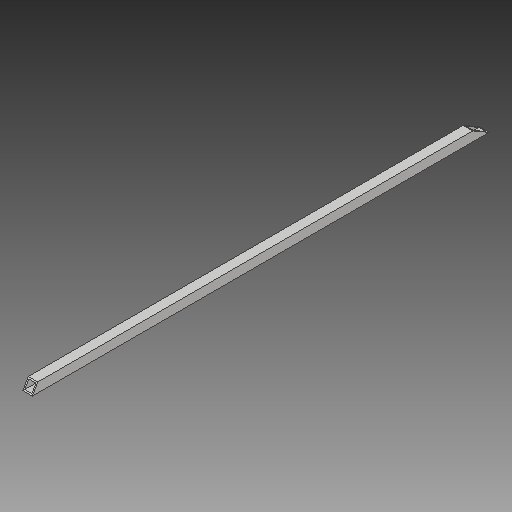
# Autodesk Inventor part: 30-60-supportBrace
Saved by Autodesk Inventor 2018.2 (Build 222227000, 227)
## iProperties
Created: 2018-02-07
Part Number: 30-60-supportBrace
Material: Generic
Document SubType Name: Modeling
Designer: steele
Density: 1 g/cm^3
Appearance: Default
Author: steele
Autodesk Inventor part; units mm, degrees
ref_plane "YZ Plane" through (0, 0, 0) normal (1, 0, 0) x (0, 1, 0)
ref_plane "XZ Plane" through (0, 0, 0) normal (0, 1, 0) x (-1, 0, 0)
ref_plane "XY Plane" through (0, 0, 0) normal (0, 0, 1) x (1, 0, 0)
sketch "Sketch1" plane through (0, 0, 0) normal (0, 0, 1) x (1, 0, 0)
  line L0 (-12.7, -12.7) -> (12.7, -12.7)
  line L1 (12.7, -12.7) -> (12.7, 12.7)
  line L2 (12.7, 12.7) -> (-12.7, 12.7)
  line L3 (-12.7, 12.7) -> (-12.7, -12.7)
  line L4 (-12.7, -12.7) -> (12.7, 12.7) construction
  line L5 (12.7, -12.7) -> (-12.7, 12.7) construction
  line L6 (-9.525, -9.525) -> (9.525, -9.525)
  line L7 (9.525, -9.525) -> (9.525, 9.525)
  line L8 (9.525, 9.525) -> (-9.525, 9.525)
  line L9 (-9.525, 9.525) -> (-9.525, -9.525)
  line L10 (-9.525, -9.525) -> (9.525, 9.525) construction
  line L11 (9.525, -9.525) -> (-9.525, 9.525) construction
  point P0 (0, 0)
  dimension "d0" = 25.4
  dimension "d1" = 3.175
  constraints: 24 end point, 4 midpoint, 4 parallel, 4 perpendicular, 2 horizontal
  measures "d0" distance of L0.start L0.end
  measures "d1" distance between parallel lines of L0 L6
extrude "Extrusion1" add sketch "Sketch1" along normal mid plane 1219.2
sketch "Sketch3" plane through (12.7, -12.7, 609.6) normal (1, 0, 0) x (0, 0, -1)
  line L0 (1219.2, 25.4) -> (0, 25.4) projected
  line L1 (0, 0) -> (1219.2, 0) projected
  line L2 (0, 25.4) -> (0, 0)
  line L3 (0, 0) -> (14.6647, 25.4)
  line L4 (1219.2, 0) -> (1219.2, 25.4)
  line L5 (1219.2, 22.225) -> (1219.2, 3.175) projected
  line L6 (1175.2059, 25.4) -> (1219.2, 0)
  point P0 (609.6, 12.7)
  dimension "d6" = 30
  dimension "d7" = 60
  constraints: 8 end point, 2 point on line, 1 collinear, 1 perpendicular
  measures "d6" angle of L2 L3
  measures "d7" angle of L4 L6
extrude "Extrusion3" cut sketch "Sketch3" against normal through all contours L4 L6 L0 | L3 L2 L0
body "Solid1"
